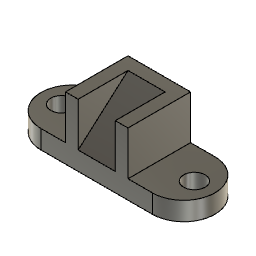
A2 (Autodesk Fusion 360 design; units mm, degrees)
Autodesk Fusion 360 part; units mm, degrees
sketch "base" plane through (0, 0, 0) normal (0, 0, 1) x (1, 0, 0)
  line L0 (0, 0) -> (1, 0)
  line L1 (1, -64) -> (0, -64)
  line L2 (0, -64) -> (0, 0)
  line L3 (0, 0) -> (114, 0)
  line L4 (114, 0) -> (114, -64)
  line L5 (0, -64) -> (114, -64)
  dimension "d1" = 64
  dimension "d2" = 114
  dimension "d3" = 64
  constraint horizontal L0
  constraint horizontal L1
  constraint vertical L2
  constraint coincident L0.start L2.end
  constraint perpendicular L3 L4
  measures "d1" distance of L0.start L1.end
  measures "d2" distance of L0.start L3.end
  measures "d3" distance of L3.end L4.end
extrude "Extrude1" add sketch "base" against normal blind 19
sketch "fillets" plane through (0, 0, -19) normal (0, 0, -1) x (1, 0, 0)
  line L0 (0, 64) -> (0, 0)
  line L1 (0, 0) -> (114, 0)
  line L2 (114, 0) -> (114, 64)
  line L3 (114, 64) -> (0, 64)
  line L4 (0, 64) -> (-32, 64)
  line L5 (-32, 64) -> (-32, 0)
  line L6 (-32, 0) -> (0, 0)
  line L7 (0, 0) -> (0, 64)
  line L8 (57, 0) -> (57, 64)
  line L9 (114, 64) -> (146, 64)
  line L10 (146, 64) -> (146, 0)
  line L11 (146, 0) -> (114, 0)
  line L12 (114, 0) -> (114, 64)
  dimension "d6" = 32
  dimension "d7" = 64
  constraint horizontal L4
  constraint vertical L5
  constraint horizontal L6
  constraint vertical L7
  constraint coincident L0.start L3.end
  constraint midpoint L1 L8.start
  constraint midpoint L3 L8.end
  constraint symmetric L0.start L8 L2.end
  constraint symmetric L4.end L8 L9.end
  constraint symmetric L5.end L8 L10.end
  constraint symmetric L0.end L8 L1.end
  measures "d6" distance of L0.start L4.end
  measures "d7" distance of L0.start L0.end
extrude "Extrude2" add sketch "fillets" against normal blind 19 contours L0 L4 L5 L6 L7 | L2 L9 L10 L11 L12
fillet "Fillet1" radius 32 4 edges at (-32, -64, -9.5) (-32, 0, -9.5) (146, -64, -9.5) (146, 0, -9.5)
sketch "holes" plane through (0, 0, 0) normal (0, 0, 1) x (-1, 0, 0)
  arc A0 (-114, 64) -> (-114, 0) centre (-114, 32) ccw
  line L0 (-114, 0) -> (0, 0)
  arc A1 (0, 0) -> (0, 64) centre (0, 32) ccw
  line L1 (0, 64) -> (-114, 64)
  line L2 (32, 32) -> (22, 32)
  line L3 (-57, 0) -> (-57, 64)
  circle A2 centre (11, 32) radius 11
  circle A3 centre (-125, 32) radius 11
  dimension "d11" = 10
  dimension "d12" = 22
  constraint midpoint A1 L2.start
  constraint horizontal L2
  constraint midpoint L0 L3.start
  constraint midpoint L1 L3.end
  constraint symmetric L3 A2 A3
  measures "d11" distance of L2.start L2.end
  measures "d12" diameter of A2
extrude "Extrude3" cut sketch "holes" against normal blind 19 contours A2 | A3
sketch "inner base" plane through (0, 0, 0) normal (0, 0, 1) x (-1, 0, 0)
  circle A0 centre (11, 32) radius 11
  circle A1 centre (-125, 32) radius 11
  arc A2 (-114, 64) -> (-114, 0) centre (-114, 32) ccw
  line L0 (-114, 0) -> (0, 0)
  arc A3 (0, 0) -> (0, 64) centre (0, 32) ccw
  line L1 (0, 64) -> (-114, 64)
  line L2 (0, 64) -> (-25, 64)
  line L3 (-25, 64) -> (-89, 64)
  line L4 (-25, 64) -> (-38, 64)
  line L5 (-25, 64) -> (-38, 64)
  line L6 (-38, 64) -> (-38, 0)
  line L7 (-38, 0) -> (-25, 0)
  line L8 (-25, 0) -> (-25, 64)
  line L9 (-57, 0) -> (-57, 64)
  line L10 (-76, 0) -> (-89, 0)
  line L11 (-89, 0) -> (-89, 64)
  line L12 (-76, 64) -> (-76, 0)
  line L13 (-89, 64) -> (-76, 64)
  line L14 (-25, 0) -> (-89, 0)
  line L15 (-89, 0) -> (-89, 13)
  line L16 (-89, 13) -> (-25, 13)
  line L17 (-25, 13) -> (-25, 0)
  dimension "d15" = 25
  dimension "d16" = 64
  dimension "d17" = 13
  dimension "d18" = 13
  constraint coincident A3.end L1.start
  constraint parallel L1 L2
  constraint parallel L1 L3
  constraint parallel L3 L4
  constraint horizontal L5
  constraint vertical L6
  constraint horizontal L7
  constraint vertical L8
  constraint coincident L0 L6.end
  constraint midpoint L0 L9.start
  constraint midpoint L3 L9.end
  constraint symmetric L2.end L9 L3.end
  constraint symmetric L4.end L9 L12.start
  constraint symmetric L6.end L9 L10.start
  constraint symmetric L7.end L9 L10.end
  constraint horizontal L14
  constraint vertical L15
  constraint horizontal L16
  constraint vertical L17
  measures "d15" distance of A3.end L2.end
  measures "d16" distance of L2.end L3.end
  measures "d17" distance of L2.end L4.end
  measures "d18" distance of L7.end L16.end
extrude "Extrude4" add sketch "inner base" along normal blind 45 contours L1 L3 L11 L12 L13 L16 | L0 L10 L11 L12 L14 L15 L16 | L0 L9 L12 L14 L16 | L0 L6 L9 L14 L16 | L1 L3 L4 L5 L6 L8 L16 | L0 L6 L7 L8 L14 L16 L17
sketch "triangle thing" plane through (25, 0, 0) normal (-1, 0, 0) x (0, -1, 0)
  line L0 (0, 0) -> (64, 0)
  line L1 (64, 0) -> (64, 45)
  line L2 (64, 45) -> (0, 45)
  line L3 (0, 45) -> (0, 0)
  line L4 (64, 0, -13) -> (13, 45, -13)
  line L5 (13, 45, -13) -> (13, 0, -13)
  line L6 (13, 0, -13) -> (64, 0, -13)
extrude "Extrude5" add sketch "triangle thing" against normal blind 38 contours L4 L5 L6 in plane through (38, 0, 0) normal (-1, 0, 0)
named bodies: "Main Body"
